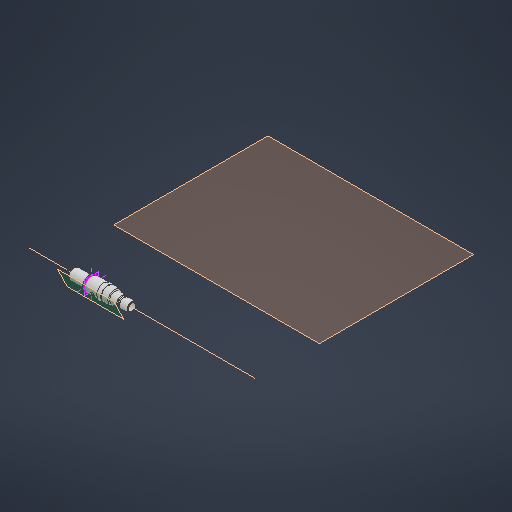
# Autodesk Inventor part: nakrętka
Saved by Autodesk Inventor 2026.1 (Build 301233020, 233B)
## iProperties
Created: 2026-02-26
Part Number: nakrętka
Material: Generic
Document SubType Name: Modeling
Designer: Jan
Density: 1 g/cm^3
Appearance: Default
Author: Jan
Autodesk Inventor part; units mm, degrees
ref_plane "YZ Plane" through (0, 0, 0) normal (1, 0, 0) x (0, 1, 0)
ref_plane "XZ Plane" through (0, 0, 0) normal (0, 1, 0) x (-1, 0, 0)
ref_plane "XY Plane" through (0, 0, 0) normal (0, 0, 1) x (1, 0, 0)
sketch "Sketch2" plane through (0, 0, 0) normal (0, 0, 1) x (1, 0, 0)
  line L0 (0, 4) -> (0.5, 4.5)
  line L1 (0, 4) -> (0, 3)
  line L2 (0.5, 4.5) -> (1.1, 4.5)
  line L3 (1.1, 4.5) -> (1.1, 4.3)
  line L4 (1.1, 4.3) -> (2.1, 4.3)
  line L5 (2.1, 4.3) -> (2.1, 4.5)
  line L6 (2.1, 4.5) -> (15.1, 4.5)
  line L7 (15.1, 4.5) -> (15.1, 5.5)
  line L8 (15.1, 5.5) -> (15.6, 6)
  line L9 (0, 3) -> (20, 3)
  line L10 (20, 3) -> (20.2, 3.2)
  line L11 (44.15, 4.5) -> (44.15, 4.3)
  line L12 (44.15, 4.3) -> (43.15, 4.3)
  line L13 (43.15, 4.3) -> (43.15, 4.5)
  line L14 (0, 0) -> (27.0854, 0) construction
  line L15 (15.6, 6) -> (16.1, 6)
  line L16 (16.1, 6) -> (16.1, 5)
  line L17 (16.1, 5) -> (17.1, 5)
  line L18 (17.1, 5) -> (17.1, 6)
  line L19 (31.9, 6) -> (31.5, 6)
  line L20 (31.5, 6) -> (31.5, 6.5)
  line L21 (31.5, 6.5) -> (28.1, 6.5)
  line L22 (28.1, 6.5) -> (28.1, 6)
  line L23 (17.1, 6) -> (28.1, 6)
  line L24 (20.2, 3.2) -> (43.9, 3.2)
  line L25 (44.15, 4.5) -> (45.15, 4.5)
  line L26 (43.15, 4.5) -> (37.9, 4.5)
  line L27 (37.15, 6) -> (31.9, 6)
  line L28 (43.9, 3.2) -> (49.9, 3.2)
  line L29 (49.9, 4) -> (45.15, 4)
  line L30 (45.15, 4) -> (45.15, 4.5)
  line L31 (49.9, 3.2) -> (51.9, 3.2)
  line L32 (51.9, 3.2) -> (51.9, 4)
  line L33 (51.9, 4) -> (49.9, 4)
  line L34 (37.9, 4.5) -> (37.15, 4.5)
  line L35 (37.15, 4.5) -> (37.15, 6)
  point P0 (1.1, 4.4)
  point P1 (15.85, 6)
  point P2 (16.6, 5)
  dimension "d3" = 4
  dimension "d8" = 1
  dimension "d9" = 0.5
  dimension "d10" = 0.5
  dimension "d11" = 0.2
  dimension "d12" = 1
  dimension "d13" = 13
  dimension "d14" = 1
  dimension "d15" = 20
  dimension "d26" = 0.2
  dimension "d27" = 0.2
  dimension "d29" = 0.5
  dimension "d30" = 0.5
  dimension "d36" = 1.1
  dimension "d37" = 4.5
  dimension "d38" = 3
  dimension "d39" = 0.5
  dimension "d40" = 1
  dimension "d41" = 1
  dimension "d60" = 0.4
  dimension "d61" = 0.5
  dimension "d62" = 3.4
  dimension "d63" = 11
  dimension "d65" = 1
  dimension "d66" = 5.25
  dimension "d83" = 6
  dimension "d84" = 0.8
  dimension "d85" = 2
  dimension "d86" = 0.75
  constraints: 72 end point, 16 horizontal, 11 perpendicular, 3 midpoint, 2 vertical, 1 parallel
  measures "d3" distance of L14.start L0.start
  measures "d8" distance of L0.start L1.end
  measures "d9" horizontal distance of L0.end L0.start
  measures "d10" horizontal distance of L0.end L0.start
  measures "d11" distance of L2.end L3.end
  measures "d12" distance of L3.end L4.end
  measures "d13" distance of L5.end L6.end
  measures "d14" distance of L6.end L7.end
  measures "d15" distance of L1.end L9.end
  measures "d26" horizontal distance of L10.end L9.end
  measures "d27" horizontal distance of L10.end L9.end
  measures "d29" horizontal distance of L8.end L7.end
  measures "d30" horizontal distance of L8.end L7.end
  measures "d36" horizontal distance of point (1.1, 4.4) L14.start
  measures "d37" distance from line of L6 L14.start
  measures "d38" distance of L1.end L14.start
  measures "d39" distance of L8.end L15.end
  measures "d40" distance of L16.end L17.end
  measures "d41" vertical distance of point (15.85, 6) point (16.6, 5)
  measures "d60" distance of L19.start L19.end
  measures "d61" distance of L19.end L20.end
  measures "d62" distance of L20.end L21.end
  measures "d63" distance of L18.end L22.end
  measures "d65" distance of L11.start L25.end
  measures "d66" distance of L13.end L26.end
  measures "d83" distance of L24.end L28.end
  measures "d84" distance of L28.end L29.start
  measures "d85" distance of L28.end L31.end
  measures "d86" distance of L26.end L34.end
revolve "Revolution1" add sketch "Sketch2" angle 360 about axis through (0, 0, 0) along (1, 0, 0)
thread "Thread1" size "M6x1" class "6H" standard "ISO Metric profile" full length
ref_plane "Work Plane1" through (51.1424, -20, -139.2633) normal (0, 1, 0) x (-1, 0, 0)
sketch "Sketch4" plane through (17.1, 0, 0) normal (-1, 0, 0) x (0, 0, 1)
  circle A0 centre (0, 0) radius 6 projected
  point P0 (0, 6)
  point P1 (6, 0)
  point P2 (0, -6.0107)
  point P3 (-6.0435, 0)
  constraints: 2 point on circle
ref_plane "Work Plane2" through (22.6, -2.6349, 5.3905) normal (0, 0.4391574, -0.8984101) x (1, 0, 0)
ref_plane "Work Plane3" through (25.4, -2.6349, 5.3905) normal (0, 0.4391574, -0.8984101) x (1, 0, 0)
sketch "Sketch7" plane through (22.6, -2.6349, 5.3905) normal (0, 0.4391574, -0.8984101) x (1, 0, 0)
  line L0 (2.6, 5) -> (0.1, 5)
  line L1 (0.1, 5) -> (0.1, -5)
  line L2 (0.1, -5) -> (2.6, -5)
  line L3 (2.6, -5) -> (2.6, 5)
  line L4 (2.6, 5) -> (0.1, -5) construction
  line L5 (0.1, 5) -> (2.6, -5) construction
  line L6 (-22.6, -4) -> (-22.6, 4) construction
  point P0 (-22.6, 0)
  point P1 (1.35, 0)
  dimension "d68" = 2.5
  dimension "d69" = 10
  dimension "d70" = 23.95
  constraints: 12 end point, 2 midpoint, 2 parallel, 1 horizontal, 1 horizontal alignment, 1 perpendicular
  measures "d68" distance of L2.end L1.end
  measures "d69" distance of L1.end L0.end
  measures "d70" distance from line of L6 point (1.35, 0)
extrude "Extrusion3" cut sketch "Sketch7" along normal blind 0.5
hole "Hole2" at (23.95, -2.6349, 5.3905) direction (0, 0.4391574, -0.8984101) diameter 1.221 depth 5.3 tip angle 118 thread size "M1.6x0.35" class "6H" standard "ISO Metric profile"
chamfer "Chamfer2" distance 0.2 angle 45 1 edges at (23.95, -1.866, 5.2076)
chamfer "Chamfer3" distance 0.3 angle 45 1 edges at (51.9, -4, 0)
body "Solid2"
